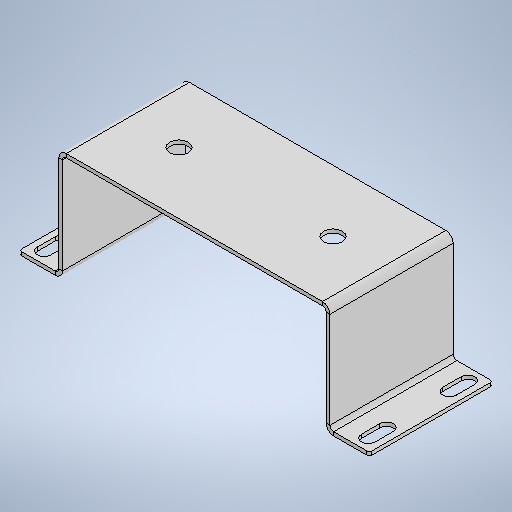
# Autodesk Inventor part: DMF Подставка ркдуктор_CPY
Saved by Autodesk Inventor 2026.2 (Build 302298010, 298A)
## iProperties
Created: 2026-06-04
Part Number: DMF Подставка ркдуктор_CPY
Material: Generic
Description: DIE16(5)|\ 90°|corrY -___°|X_____|bom___
Document SubType Name: Sheet Metal
Designer: admin
Stock Number: МОО 305 шпангоут борт
Mass: 1762.25 g
Surface Area: 2283.33 cm^2
Volume: 220.281 cm^3
Density: 1 g/cm^3
Flat Pattern Width: 10 cm
Flat Pattern Length: 44.9143 cm
Flat Pattern Area: 449.143 cm^2
Sheet Metal Rule: Default
Sheet Metal Width: 100,000 mm
Sheet Metal Length: 449,143 mm
Sheet Metal Area: 44914,336 mm^2
Appearance: Default
Author: admin
Autodesk Inventor part; units mm, degrees
ref_plane "YZ Plane" through (0, 0, 0) normal (1, 0, 0) x (0, 1, 0)
ref_plane "XZ Plane" through (0, 0, 0) normal (0, 1, 0) x (-1, 0, 0)
ref_plane "XY Plane" through (0, 0, 0) normal (0, 0, 1) x (1, 0, 0)
sketch "Sketch1" plane through (0, 0, 0) normal (0, 0, 1) x (1, 0, 0)
  line L0 (-110, -50) -> (110, -50)
  line L1 (110, -50) -> (110, 50)
  line L2 (110, 50) -> (-110, 50)
  line L3 (-110, 50) -> (-110, -50)
  line L4 (-110, -50) -> (110, 50) construction
  circle A0 centre (-62.5, 0) radius 7.5
  circle A1 centre (62.5, 0) radius 7.5
  line L5 (0, 50) -> (0, -50) construction
  line L6 (-110, 0) -> (110, 0) construction
  line L7 (-70, 0) -> (-55, 0) construction
  point P0 (0, 0)
  dimension "d154" = 220
  dimension "d155" = 100
  dimension "d159" = 15
  dimension "d160" = 125
  dimension "d190" = 15
  measures "d154" distance of L1.end L2.end
  measures "d155" distance of L0.end L1.end
  measures "d159" diameter of A0
  measures "d160" distance of A1.centre A0.centre
  measures "d190" distance of L7.start L7.end
extrude "Plate5" add sketch "Sketch1" along normal blind 3
sketch "Sketch7" plane through (-107, 50, 3) normal (-1, 0, 0) x (0, -1, 0)
  line L0 (100, 0) -> (0, 0)
  line L1 (0, 0) -> (0, -90)
  line L2 (0, -90) -> (100, -90)
  line L3 (100, -90) -> (100, 0)
  constraints: 6 end point, 1 horizontal, 1 perpendicular, 1 vertical
edge flange "Flange3" height 90 angle 90 thickness 3 bend radius 3 thickness toward (-1, 0, 0) relief tear relief width 3 relief depth 1.5 corner gap 3 corner form 0 edges at (-110, 0, 0) (110, 0, 0) wall of the first edge with corners at (-107, -50, 3) (-107, 50, 3) (-107, 50, -87) (-107, -50, -87)
bend "Bend3"
corner "Corner3"
sketch "Sketch8" plane through (-107, -50, -84) normal (0, 0, -1) x (-1, 0, 0)
  line L0 (0, 100) -> (0, 0)
  line L1 (0, 0) -> (35, 0)
  line L2 (35, 0) -> (35, 100)
  line L3 (35, 100) -> (0, 100)
  constraints: 6 end point, 1 horizontal, 1 perpendicular, 1 vertical
edge flange "Flange4" height 35 angle 90 thickness 3 bend radius 3 thickness toward (0, 0, -1) relief tear relief width 3 relief depth 1.5 corner gap 3 corner form 0 edges at (-110, 0, -87) (110, 0, -87) wall of the first edge with corners at (-107, 50, -84) (-107, -50, -84) (-142, -50, -84) (-142, 50, -84)
bend "Bend4"
corner "Corner4"
sketch "Sketch9" plane through (-142, -50, -87) normal (0, 0, -1) x (-1, 0, 0)
  line L0 (-10.5, 9.5) -> (-10.5, 24.5) construction
  line L1 (-5, 9.5) -> (-5, 24.5)
  line L2 (-16, 24.5) -> (-16, 9.5)
  arc A0 (-16, 9.5) -> (-5, 9.5) centre (-10.5, 9.5) ccw
  arc A1 (-5, 24.5) -> (-16, 24.5) centre (-10.5, 24.5) ccw
  line L3 (-10.5, 75.5) -> (-10.5, 90.5) construction
  line L4 (-5, 75.5) -> (-5, 90.5)
  line L5 (-16, 90.5) -> (-16, 75.5)
  arc A2 (-16, 75.5) -> (-5, 75.5) centre (-10.5, 75.5) ccw
  arc A3 (-5, 90.5) -> (-16, 90.5) centre (-10.5, 90.5) ccw
  line L6 (0, 100) -> (0, 0) projected
  line L7 (0, 50) -> (-19.5858, 50)
  point P0 (-142, 50)
  point P1 (-10.5, 17)
  point P2 (-10.5, 83)
  point P3 (-10.5, 30)
  point P4 (-10.5, 70)
  dimension "d182" = 11
  dimension "d183" = 15
  dimension "d184" = 5
  dimension "d186" = 40
  constraints: 18 end point, 10 point on circle, 8 tangent, 4 centre point, 3 midpoint, 2 collinear, 2 parallel, 2 vertical, 1 equal radius, 1 horizontal, 1 symmetric about line
  measures "d182" distance between parallel lines of L5 L4
  measures "d183" distance of L3.start L3.end
  measures "d184" distance between parallel lines of L4 L6
  measures "d186" distance of point (-10.5, 30) point (-10.5, 70)
extrude "Cut1" cut sketch "Sketch9" against normal blind 3
mirror "Mirror1" about plane through (0, 0, 0) normal (1, 0, 0) of "Cut1"
fillet "Corner Round2" radius 2 4 edges at (-142, 50, -85.5) (-142, -50, -85.5) (142, -50, -85.5) (142, 50, -85.5)
body "Solid3"
